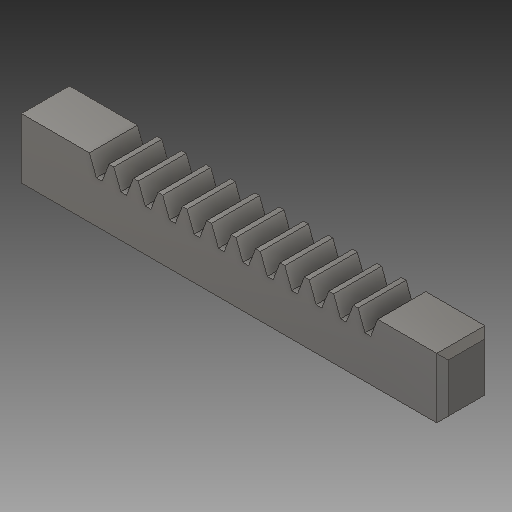
# Autodesk Inventor part: Gear Rack
Saved by Autodesk Inventor 2018 (Build 220112000, 112)
## iProperties
Created: 2017-12-21
Part Number: Gear Rack
Material: Stainless Steel
Document SubType Name: Modeling
Designer: 232963
Density: 8 g/cm^3
Appearance: Semi-Polished
Author: 232963
Autodesk Inventor part; units mm, degrees
ref_plane "YZ Plane" through (0, 0, 0) normal (1, 0, 0) x (0, 1, 0)
ref_plane "XZ Plane" through (0, 0, 0) normal (0, 1, 0) x (-1, 0, 0)
ref_plane "XY Plane" through (0, 0, 0) normal (0, 0, 1) x (1, 0, 0)
sketch "Sketch1" plane through (0, 0, 0) normal (0, 0, 1) x (1, 0, 0)
  line L0 (-5.1073, 0) -> (106.1447, 0)
  line L1 (106.1447, 0) -> (106.1447, 15.875)
  line L2 (106.1447, 15.875) -> (-5.1073, 15.875)
  line L3 (-5.1073, 15.875) -> (-5.1073, 0)
  point P0 (0, 0)
  dimension "d0" = 111.252
  dimension "d1" = 15.875
  constraints: 8 end point, 2 parallel, 1 horizontal, 1 perpendicular
  measures "d0" distance of L2.end L1.end
  measures "d1" distance of L1.end L0.end
extrude "Extrusion1" add sketch "Sketch1" along normal blind 12.7
sketch "Sketch2" plane through (0, 0, 12.7) normal (0, 0, 1) x (1, 0, 0)
  line L0 (106.1447, 15.875) -> (-5.1073, 15.875) projected
  line L1 (12.8596, 15.875) -> (14.6926, 11.0998)
  line L2 (-5.1073, 0) -> (106.1447, 0) projected
  line L3 (14.6926, 11.0998) -> (16.2166, 11.0998)
  line L4 (16.2166, 11.0998) -> (18.0497, 15.875)
  point P0 (0, 0)
  dimension "d4" = 17.9669
  dimension "d5" = 11.0998
  dimension "d6" = 11.0998
  dimension "d10" = 42
  dimension "d11" = 1.524
  constraints: 6 end point, 2 point on line, 1 horizontal
  measures "d4" distance of L1.start L0.end
  measures "d5" distance from line of L2 L1.end
  measures "d6" distance from line of L2 L3.end
  measures "d10" angle of L4 L1
  measures "d11" distance of L1.end L3.end
extrude "Extrusion2" cut sketch "Sketch2" against normal blind 12.7
pattern_linear "Rectangular Pattern1" count 12 spacing 6.4516 along (1, 0, 0) of "Extrusion2"
chamfer "Chamfer1" distance 1.524 angle 45 4 edges at (106.1447, 7.9375, 12.7) (106.1447, 15.875, 6.35) (106.1447, 7.9375, 0) (106.1447, 0, 6.35)
sketch "Sketch3" plane through (-5.1073, 0, 0) normal (-1, 0, 0) x (0, 0, 1)
  circle A0 centre (6.35, 7.9248) radius 3.175
  line L0 (0, 15.875) -> (12.7, 15.875) projected
  line L1 (0, 15.875) -> (0, 0) projected
  dimension "d20" = 6.35
  dimension "d21" = 7.9502
  dimension "d22" = 6.35
  constraints: 1 centre point
  measures "d20" diameter of A0
  measures "d21" distance from line of L0 A0.centre
  measures "d22" distance from line of L1 A0.centre
extrude "Extrusion3" cut sketch "Sketch3" against normal blind 15.875
body "Solid1"
